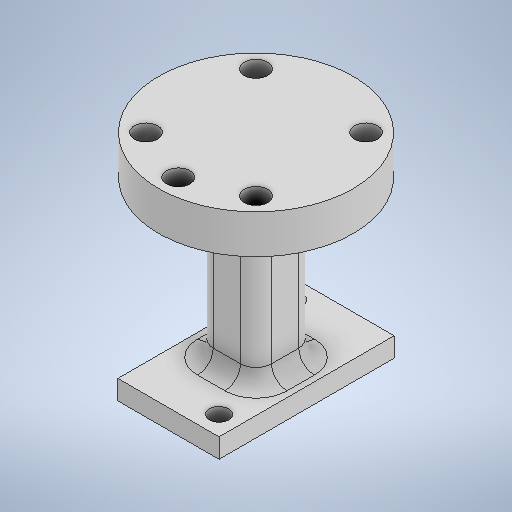
# Autodesk Inventor part: Flange
Saved by Autodesk Inventor 2025 (Build 290162000, 162)
## iProperties
Created: 2025-07-10
Part Number: Flange
Material: Genérico
Document SubType Name: Modeling
Designer: acer
Density: 1 g/cm^3
Appearance: Valor por defecto
Author: acer
Autodesk Inventor part; units mm, degrees
ref_plane "YZ Plane" through (0, 0, 0) normal (1, 0, 0) x (0, 1, 0)
ref_plane "XZ Plane" through (0, 0, 0) normal (0, 1, 0) x (-1, 0, 0)
ref_plane "XY Plane" through (0, 0, 0) normal (0, 0, 1) x (1, 0, 0)
sketch "Boceto1" plane through (0, 0, 0) normal (0, 1, 0) x (-1, 0, 0)
  line L0 (0, 0) -> (26, 0)
  line L1 (26, 0) -> (26, -45)
  line L2 (26, -45) -> (0, -45)
  line L3 (0, -45) -> (0, 0)
  dimension "d0" = 26
  dimension "d1" = 45
  constraints: 8 end point, 2 parallel, 1 horizontal, 1 perpendicular
  measures "d0" distance of L1.end L2.end
  measures "d1" distance of L0.end L1.end
extrude "Extrusión1" add sketch "Boceto1" along normal blind 5
sketch "Boceto2" plane through (0, 5, 0) normal (0, 1, 0) x (1, 0, 0)
  line L0 (-26, 0) -> (0, 0) projected
  line L1 (0, 0) -> (-5, 0)
  line L2 (0, 45) -> (-26, 45) projected
  line L3 (-26, 45) -> (-21, 45)
  line L4 (0, 45) -> (0, 40)
  line L5 (0, 0) -> (0, 45) projected
  line L6 (0, 0) -> (0, 5)
  line L7 (-26, 45) -> (-26, 0) projected
  circle A0 centre (-21, 40) radius 2.5
  circle A1 centre (-5, 5) radius 2.5
  dimension "d4" = 5
  dimension "d6" = 5
  dimension "d7" = 5
  dimension "d9" = 5
  dimension "d10" = 5
  constraints: 8 end point, 4 point on line, 2 centre point
  measures "d4" distance of L0.end L1.end
  measures "d6" distance of L2.end L3.end
  measures "d7" distance of L2.start L4.end
  measures "d9" diameter of A0
  measures "d10" diameter of A1
extrude "Extrusión2" cut sketch "Boceto2" against normal blind 5 contours A0 | A1
sketch "Boceto3" plane through (0, 5, 0) normal (0, 1, 0) x (1, 0, 0)
  line L0 (0, 0) -> (0, 45) projected
  line L1 (0, 45) -> (0, 37.5)
  line L2 (0, 45) -> (0, 30)
  line L3 (0, 0) -> (0, 15)
  line L4 (-5.5, 15) -> (-20.5, 15)
  line L5 (-20.5, 15) -> (-20.5, 30)
  line L6 (-20.5, 30) -> (-5.5, 30)
  line L7 (-5.5, 30) -> (-5.5, 15)
  constraints: 14 end point, 3 point on line, 2 perpendicular, 1 vertical
extrude "Extrusión3" add sketch "Boceto3" along normal blind 40
sketch "Boceto4" plane through (0, 45, 0) normal (0, 1, 0) x (1, 0, 0)
  line L0 (-5.5, 30) -> (-20.5, 30) projected
  line L1 (-20.5, 30) -> (-20.5, 15) projected
  line L2 (-20.5, 30) -> (-20.5, 15)
  line L3 (-5.5, 15) -> (-5.5, 30) projected
  circle A0 centre (-13, 22.5) radius 25
  point P0 (0, 0)
  constraints: 2 end point, 1 centre point, 1 collinear
extrude "Extrusión4" add sketch "Boceto4" along normal blind 10
fillet "Empalme1" radius 4 12 edges at (-13, 45, -30) (-5.5, 25, -30) (-5.5, 45, -22.5) (-5.5, 25, -15) (-20.5, 25, -30) (-20.5, 25, -15) (-13, 45, -15) (-20.5, 45, -22.5) (-20.5, 5, -22.5) (-13, 5, -15) (-13, 5, -30) (-5.5, 5, -22.5)
sketch "Boceto6" plane through (-13, 55, -22.5) normal (0, 1, 0) x (1, 0, 0)
  circle A0 centre (0, -20) radius 3
  line L0 (0, 0) -> (31.4027, 0) construction
  line L1 (0, 0) -> (28.2843, 0) construction
  circle A1 centre (14.1421, 14.1421) radius 3
  circle A2 centre (-14.1421, 14.1421) radius 3
  circle A3 centre (-14.1421, -14.1421) radius 3
  circle A4 centre (14.1421, -14.1421) radius 3
  point P0 (13, -22.5)
  dimension "d27" = 6
  dimension "d32" = 6
  dimension "d33" = 6
  dimension "d34" = 6
  dimension "d35" = 6
  constraints: 5 centre point, 4 end point, 2 horizontal
  measures "d27" diameter of A0
  measures "d32" diameter of A1
  measures "d33" diameter of A2
  measures "d34" diameter of A3
  measures "d35" diameter of A4
extrude "Extrusión5" cut sketch "Boceto6" against normal blind 10
